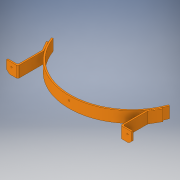
# Autodesk Inventor part: Half moon catch
Saved by Autodesk Inventor 2017 (Build 210142000, 142)
## iProperties
Created: 2017-01-15
Part Number: Half moon catch
Material: Generic
Document SubType Name: Modeling
Designer: Ben
Density: 1 g/cm^3
Appearance: Orange
Author: Ben
Autodesk Inventor part; units mm, degrees
ref_plane "YZ Plane" through (0, 0, 0) normal (1, 0, 0) x (0, 1, 0)
ref_plane "XZ Plane" through (0, 0, 0) normal (0, 1, 0) x (-1, 0, 0)
ref_plane "XY Plane" through (0, 0, 0) normal (0, 0, 1) x (1, 0, 0)
sketch "Sketch1" plane through (0, 0, 0) normal (0, 1, 0) x (-1, 0, 0)
  arc A0 (131.2751, 47.7802) -> (-131.2751, 47.7802) centre (0, 0) ccw
  arc A1 (134.2586, 48.8661) -> (-134.2586, 48.8661) centre (0, 0) ccw
  line L0 (150.3938, 142.875) -> (-175.7852, 142.875) construction
  line L1 (0, 0) -> (131.2751, 47.7802) construction
  line L2 (0, 0) -> (-131.2751, 47.7802) construction
  line L3 (0, 0) -> (0, 139.7) construction
  line L4 (-131.2751, 47.7802) -> (-134.2586, 48.8661)
  line L5 (131.2751, 47.7802) -> (134.2586, 48.8661)
  line L6 (130.0834, 60.439) -> (116.958, 83.1728)
  line L7 (116.958, 83.1728) -> (116.958, 142.875)
  line L8 (116.958, 142.875) -> (142.358, 142.875)
  line L9 (142.358, 139.7) -> (142.358, 142.875)
  line L10 (142.358, 139.7) -> (120.133, 139.7)
  line L11 (120.133, 139.7) -> (120.133, 84.0235)
  line L12 (120.133, 84.0235) -> (132.833, 62.0265)
  line L13 (132.833, 62.0265) -> (130.0834, 60.439)
  line L14 (120.133, 139.7) -> (116.958, 139.7) construction
  line L15 (123.7334, 71.4375) -> (126.483, 73.025) construction
  line L16 (-130.0834, 60.439) -> (-116.958, 83.1728)
  line L17 (-116.958, 83.1728) -> (-116.958, 142.875)
  line L18 (-116.958, 142.875) -> (-142.358, 142.875)
  line L19 (-142.358, 139.7) -> (-142.358, 142.875)
  line L20 (-142.358, 139.7) -> (-120.133, 139.7)
  line L21 (-120.133, 139.7) -> (-120.133, 84.0235)
  line L22 (-120.133, 84.0235) -> (-132.833, 62.0265)
  line L23 (-132.833, 62.0265) -> (-130.0834, 60.439)
  dimension "d1" = 3.175
  dimension "d4" = 279.4
  dimension "d6" = 140
  dimension "d7" = 3.175
  dimension "d8" = 25.4
  dimension "d9" = 30
  dimension "d10" = 25.4
  constraints: 48 end point, 8 symmetric about line, 6 perpendicular, 6 point on circle, 4 coincident, 4 point on line, 2 centre point, 2 collinear, 2 equal length, 2 horizontal, 2 tangent, 1 midpoint, 1 parallel, 1 vertical
  measures "d1" distance of L5.end L1.end
  measures "d4" diameter of A0
  measures "d6" angle of L1 L2
  measures "d7" distance of L9.start L8.end
  measures "d8" distance of L7.end L8.end
  measures "d9" angle of L7 L6
  measures "d10" distance of L11.end L12.end
extrude "Extrusion1" add sketch "Sketch1" along normal blind 25.4
fillet "Fillet1" radius 3.175 4 edges at (-120.133, 12.7, 139.7) (-116.958, 12.7, 142.875) (116.958, 12.7, 142.875) (120.133, 12.7, 139.7)
sketch "Sketch2" plane through (-142.358, 0, 142.875) normal (0, 0, 1) x (1, 0, 0)
  line L0 (142.358, 0) -> (142.358, 6.35) construction
  line L1 (11.083, 0) -> (11.083, 25.4) construction
  line L2 (11.083, 25.4) -> (11.083, 6.35) construction
  line L3 (275.191, 0) -> (275.191, 25.4) construction
  line L4 (275.191, 25.4) -> (275.191, 6.35) construction
  circle A0 centre (11.083, 15.875) radius 1.5875
  circle A1 centre (142.358, 15.875) radius 1.5875
  circle A2 centre (275.191, 15.875) radius 1.5875
  line L5 (275.191, 6.35) -> (11.083, 6.35) construction
  line L6 (11.083, 6.35) -> (11.083, 0) construction
  line L7 (275.191, 6.35) -> (275.191, 0) construction
  line L8 (142.358, 6.35) -> (142.358, 25.4) construction
  line L9 (266.0914, 25.4) -> (18.6246, 25.4) construction
  dimension "d13" = 3.175
  dimension "d16" = 19.05
  constraints: 14 end point, 4 collinear, 4 midpoint, 3 centre point, 2 coincident, 2 equal radius, 2 point on line, 2 vertical, 1 horizontal
  measures "d13" diameter of A2
  measures "d16" distance from line of L1.end L5
extrude "Extrusion2" cut sketch "Sketch2" against normal blind 25.4
chamfer "Chamfer1" distance 6.35 angle 45 2 edges at (142.358, 0, 141.2875) (-142.358, 0, 141.2875)
fillet "Fillet2" radius 6.35 2 edges at (-136.008, 0, 141.2875) (136.008, 0, 141.2875)
body "Solid1"
